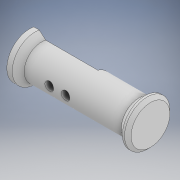
# Autodesk Inventor part: FS_ShaftV3
Saved by Autodesk Inventor 2020 (Build 240168000, 168)
## iProperties
Created: 2020-08-20
Part Number: FS_ShaftV3
Material: Generic
Document SubType Name: Modeling
Designer: Theo Cominotto
Density: 1 g/cm^3
Appearance: Default
Author: Theo Cominotto
Autodesk Inventor part; units mm, degrees
ref_plane "YZ Plane" through (0, 0, 0) normal (1, 0, 0) x (0, 1, 0)
ref_plane "XZ Plane" through (0, 0, 0) normal (0, 1, 0) x (-1, 0, 0)
sketch "Sketch1" plane through (0, 0, 0) normal (0, 0, 1) x (1, 0, 0)
  line L0 (0, -4.2) -> (0, 25.2) construction
  line L1 (-78.4, 0) -> (78.4, 0) construction
  line L2 (-45, 16) -> (45, 16)
  line L3 (45, 16) -> (45, 0)
  line L4 (45, 0) -> (-45, 0)
  line L5 (-45, 0) -> (-45, 16)
  line L6 (-45, 0) -> (-51, 0)
  line L7 (-51, 0) -> (-51, 21)
  line L8 (-51, 21) -> (-45, 16)
  line L9 (-51, 21) -> (-56, 21)
  line L10 (-56, 21) -> (-56, 0)
  line L11 (-56, 0) -> (-51, 0)
  line L12 (-51, 0) -> (-51, 21)
  line L13 (45, 0) -> (45, 16)
  line L14 (45, 0) -> (51, 0)
  line L15 (51, 0) -> (51, 21)
  line L16 (51, 21) -> (45, 16)
  line L17 (51, 21) -> (56, 21)
  line L18 (56, 21) -> (56, 0)
  line L19 (56, 0) -> (51, 0)
  line L20 (51, 0) -> (51, 21)
  point P0 (0, 0)
  dimension "d1" = 90
  dimension "d3" = 6
  dimension "d4" = 5
  dimension "d6" = 5
  dimension "d7" = 16
  dimension "d9" = 11
  constraints: 38 end point, 5 symmetric about line, 4 parallel, 2 horizontal, 2 perpendicular, 2 point on line, 1 collinear, 1 vertical, 1 other
  measures "d1" distance of L2.start L2.end
  measures "d3" distance between parallel lines of L5 L7
  measures "d4" distance of L7.end L9.end
  measures "d6" distance between parallel lines of L9 L2
  measures "d7" distance of L4.end L2.start
  measures "d9" distance between parallel lines of L5 L10
revolve "Revolution1" add sketch "Sketch1" angle 360 about axis through (-10, 0, 0) along (1, 0, 0)
sketch "Sketch2" plane through (-56, 0, 0) normal (-1, 0, 0) x (0, 0, 1)
  line L0 (-30.6, 0) -> (29.6, 0) construction
  line L1 (-4, 20.6155) -> (-21, 20.6155)
  line L2 (-21, 20.6155) -> (-21, -20.6155)
  line L3 (-21, -20.6155) -> (-4, -20.6155)
  line L4 (-4, -20.6155) -> (-4, 20.6155)
  circle A0 centre (0, 0) radius 16 construction
  circle A1 centre (0, 0) radius 16 construction
  circle A2 centre (0, 0) radius 16 construction
  line L5 (0, 0) -> (16, 0) construction
  circle A3 centre (0, 0) radius 16 construction
  circle A4 centre (0, 0) radius 21 construction
  dimension "d8" = 20
  constraints: 10 end point, 2 parallel, 2 point on circle, 1 horizontal, 1 horizontal alignment, 1 perpendicular, 1 point on line, 1 tangent, 1 other
  measures "d8" distance from line of L5.end L4
extrude "Extrusion1" cut sketch "Sketch2" against normal blind 59.25
sketch "Sketch3" plane through (-56, -20.6155, -4) normal (0, 0, -1) x (-1, 0, 0)
  line L0 (0, 41.6155) -> (0, -0.3845) construction
  line L1 (0, 20.6155) -> (-59.25, 20.6155) construction
  line L2 (-59.25, 36.1075) -> (-59.25, 5.1236) construction
  circle A0 centre (-34.25, 20.6155) radius 2.15
  circle A1 centre (-49.25, 20.6155) radius 2.15
  line L3 (-34.25, 20.6155) -> (-49.25, 20.6155) construction
  line L4 (-11, 36.6155) -> (-11, 4.6155) construction
  line L5 (-11, 4.6155) -> (-11, 36.6155) construction
  line L6 (-5, 41.6155) -> (-11, 36.6155) construction
  line L7 (-11, 5.1236) -> (-59.25, 5.1236) construction
  line L8 (-56.25, 5.1236) -> (-56.25, 36.1075) construction
  line L9 (-59.25, 36.1075) -> (-11, 36.1075) construction
  point P0 (-56, 20.6155)
  point P1 (0, 41.2311)
  point P2 (0, 0)
  point P3 (-41.75, 20.6155)
  dimension "d14" = 4.3
  dimension "d16" = 15
  dimension "d18" = 4.3
  dimension "d21" = 3
  dimension "d22" = 14.5
  constraints: 8 end point, 5 point on line, 3 midpoint, 2 centre point, 2 vertical, 1 equal radius, 1 horizontal
  measures "d14" diameter of A1
  measures "d16" distance of L3.end L3.start
  measures "d18" diameter of A0
  measures "d21" distance from line of L1.end L8
  measures "d22" distance from line of L8 point (-41.75, 20.616)
extrude "Extrusion2" cut sketch "Sketch3" against normal up to surface
ref_plane "Work Plane1" through (-56, -20.6155, 4) normal (0, 0, -1) x (-1, 0, 0)
sketch "Sketch4" plane through (-56, -20.6155, 4) normal (0, 0, -1) x (-1, 0, 0)
  circle A0 centre (-34.25, 20.6155) radius 2.15 projected
  circle A1 centre (-34.25, 20.6155) radius 4
  circle A2 centre (-49.25, 20.6155) radius 2.15 projected
  circle A3 centre (-49.25, 20.6155) radius 4
  point P0 (-56, 20.6155)
  dimension "d24" = 8
  dimension "d25" = 8
  constraints: 2 centre point, 2 coincident
  measures "d24" diameter of A1
  measures "d25" diameter of A3
extrude "Extrusion3" cut sketch "Sketch4" against normal up to surface contours A0 | A1 | A2 | A3
chamfer "Chamfer1" distance 3 angle 45 1 edges at (56, -21, 0)
equation "\"d8\" = ShaftH"
equation "\"d10\" = d92 + d9 + LCClearance"
equation "\"d21\" = LCClearance"
equation "\"d26\" = d92 + d9 + LCClearance"
equation "\"ShaftH\" = 20"
equation "\"WallT\" = 3"
equation "\"SpoolOffset\" = 8"
equation "\"BottomT\" = 4"
equation "\"WallH\" = 45"
equation "\"ShaftL\" = 81"
equation "\"LCClearance\" = 3"
equation "\"d92\" = 45.25"
body "Solid1"
